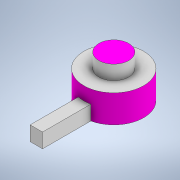
# Autodesk Inventor part: Camara
Saved by Autodesk Inventor 2021 (Build 250183000, 183)
## iProperties
Created: 2021-02-21
Part Number: Camara
Material: Generic
Document SubType Name: Modeling
Designer: deuts
Density: 1 g/cm^3
Appearance: Default
Author: deuts
Autodesk Inventor part; units mm, degrees
ref_plane "YZ Plane" through (0, 0, 0) normal (1, 0, 0) x (0, 1, 0)
ref_plane "XZ Plane" through (0, 0, 0) normal (0, 1, 0) x (-1, 0, 0)
sketch "Sketch1" plane through (0, 0, 0) normal (0, 1, 0) x (-1, 0, 0)
  circle A0 centre (0, 0) radius 30.75
  dimension "d0" = 61.5
  constraints: 1 centre point, 1 coincident
  measures "d0" diameter of A0
extrude "Extrusion1" add sketch "Sketch1" along normal blind 43.3
ref_plane "Work Plane1" through (0, 0, 30.75) normal (0, 0, 1) x (1, 0, 0)
sketch "Sketch2" plane through (0, 0, 30.75) normal (0, 0, 1) x (1, 0, 0)
  line L0 (30.75, 0) -> (-30.75, 0) projected
  line L1 (6.4, 15) -> (-6.4, 15)
  line L2 (-6.4, 15) -> (-6.4, 0)
  line L3 (-6.4, 0) -> (6.4, 0)
  line L4 (6.4, 0) -> (6.4, 15)
  constraints: 8 end point, 2 parallel, 1 horizontal, 1 perpendicular, 1 point on line
extrude "Extrusion2" add sketch "Sketch2" along normal blind 49
sketch "Sketch3" plane through (0, 0, 30.75) normal (0, 0, -1) x (-1, 0, 0)
  line L0 (6.4, 15) -> (6.4, 0) projected
  line L1 (-6.4, 0) -> (-6.4, 15) projected
  line L2 (6.4, 0) -> (-6.4, 0)
  line L3 (-6.4, 0) -> (-6.4, 15)
  line L4 (-6.4, 15) -> (6.4, 15)
  line L5 (6.4, 15) -> (6.4, 0)
  point P0 (0, 0)
  constraints: 8 end point, 2 parallel, 1 horizontal, 1 perpendicular
extrude "Extrusion3" add sketch "Sketch3" along normal blind 5
sketch "Sketch4" plane through (0, 43.3, 0) normal (0, 1, 0) x (1, 0, 0)
  circle A0 centre (0, 0) radius 15.35
  circle A1 centre (0, 0) radius 30.75
  dimension "d10" = 30.7
  constraints: 2 centre point, 2 coincident
  measures "d10" diameter of A0
extrude "Extrusion4" cut sketch "Sketch4" against normal blind 14.7
body "Solid1"
